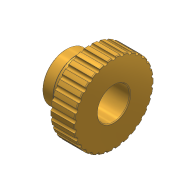
# Autodesk Inventor part: Press
Saved by Autodesk Inventor 2016 (Build 200138000, 138)
## iProperties
Created: 2020-10-21
Part Number: Press
Material: Generic
Document SubType Name: Modeling
Designer: extract
Density: 1 g/cm^3
Appearance: Default
Author: extract
Autodesk Inventor part; units mm, degrees
ref_plane "YZ Plane" through (0, 0, 0) normal (1, 0, 0) x (0, 1, 0)
ref_plane "XZ Plane" through (0, 0, 0) normal (0, 1, 0) x (-1, 0, 0)
ref_plane "XY Plane" through (0, 0, 0) normal (0, 0, 1) x (1, 0, 0)
sketch "Sketch1" plane through (0, 0, 0) normal (0, 1, 0) x (-1, 0, 0)
  arc A0 (4.6007, 3.1261) -> (6.2268, 3) centre (5.5398, 4.6888) ccw
  line L0 (6.2268, 3) -> (7.6007, 3)
  line L1 (7.6007, 3) -> (7.6007, 2)
  line L2 (7.6007, 2) -> (1.6007, 2)
  line L3 (4.6007, 3.1261) -> (4.6007, 5)
  line L4 (4.6007, 5) -> (1.6007, 5)
  line L5 (1.6007, 5) -> (1.6007, 2)
  line L6 (-1.5201, 0) -> (9.1208, 0) projected
  line L7 (6.2268, 3) -> (4.8528, 3) construction
  point P0 (0, 0)
  dimension "d0" = 2
  dimension "d1" = 3
  dimension "d2" = 5
  dimension "d3" = 6
  dimension "d10" = 3
  constraints: 14 end point, 4 perpendicular, 3 point on circle, 2 horizontal, 1 centre point, 1 collinear, 1 vertical
  measures "d0" distance between parallel lines of L6 L2
  measures "d1" distance between parallel lines of L6 L0
  measures "d2" distance between parallel lines of L6 L4
  measures "d3" distance between parallel lines of L5 L1
  measures "d10" distance of L3.end L4.end
revolve "Revolution1" add sketch "Sketch1" angle 360 about axis through (0, 0, 0) along (-1, 0, 0)
sketch "Sketch2" plane through (-1.6007, 0, 0) normal (1, 0, 0) x (0, 0, -1)
  circle A0 centre (0, 0) radius 5 projected
  circle A1 centre (-5, 0) radius 0.25
  dimension "d14" = 0.5
  constraints: 1 centre point, 1 horizontal alignment, 1 other
  measures "d14" diameter of A1
extrude "Extrusion1" cut sketch "Sketch2" against normal blind 10 contours A1 A0 | A0 A1 picked at (-4.9162, 0) picked at (-5.0822, 0.0102)
pattern_circular "Circular Pattern1" count 30 over 360 about axis through (-4.6007, 0, 0) along (-1, 0, 0) of "Extrusion1"
fillet "Fillet1" radius 0.1 65 edges at (-4.6007, 0, -3.1261) (-4.6007, -0.5226, 4.9726) (-4.6007, -1.5451, 4.7553) (-4.6007, -2.5, 4.3301) (-4.6007, -3.3457, 3.7157) (-4.6007, -4.0451, 2.9389) (-4.6007, -4.5677, 2.0337) (-4.6007, -4.8907, 1.0396) (-4.6007, -5, 0) (-4.6007, -4.8907, -1.0396) (-4.6007, -4.5677, -2.0337) (-4.6007, 0.5226, 4.9726) (-4.6007, -4.0451, -2.9389) (-4.6007, -3.3457, -3.7157) (-4.6007, -2.5, -4.3301) (-4.6007, -1.5451, -4.7553) (-4.6007, 1.5451, 4.7553) (-4.6007, 2.5, 4.3301) (-4.6007, 3.3457, 3.7157) (-4.6007, 4.0451, 2.9389) (-4.6007, 4.5677, 2.0337) (-4.6007, 4.8907, 1.0396) (-4.6007, 5, 0) (-4.6007, 4.8907, -1.0396) (-4.6007, 4.5677, -2.0337) (-4.6007, 4.0451, -2.9389) (-4.6007, 3.3457, -3.7157) (-4.6007, 2.5, -4.3301) (-4.6007, 1.5451, -4.7553) (-4.6007, 0.5226, -4.9726) (-4.6007, -0.5226, -4.9726) (-1.6007, -0.5226, 4.9726) (-1.6007, -1.5451, 4.7553) (-1.6007, -2.5, 4.3301) (-1.6007, -3.3457, 3.7157) (-1.6007, -4.0451, 2.9389) (-1.6007, -4.5677, 2.0337) (-1.6007, -4.8907, 1.0396) (-1.6007, -5, 0) (-1.6007, -4.8907, -1.0396) (-1.6007, 0.5226, 4.9726) (-1.6007, -4.5677, -2.0337) (-1.6007, -4.0451, -2.9389) (-1.6007, -3.3457, -3.7157) (-1.6007, -2.5, -4.3301) (-1.6007, -1.5451, -4.7553) (-1.6007, 1.5451, 4.7553) (-1.6007, 2.5, 4.3301) (-1.6007, 3.3457, 3.7157) (-1.6007, 4.0451, 2.9389) (-1.6007, 4.5677, 2.0337) (-1.6007, 4.8907, 1.0396) (-1.6007, 5, 0) (-1.6007, 4.8907, -1.0396) (-1.6007, 4.5677, -2.0337) (-1.6007, 4.0451, -2.9389) (-1.6007, 3.3457, -3.7157) (-1.6007, 2.5, -4.3301) (-1.6007, 1.5451, -4.7553) (-1.6007, 0.5226, -4.9726) (-1.6007, -0.5226, -4.9726) (-6.2268, 0, -3) (-7.6007, 0, -3) (-7.6007, 0, -2) (-1.6007, 0, -2)
body "Solid1"
